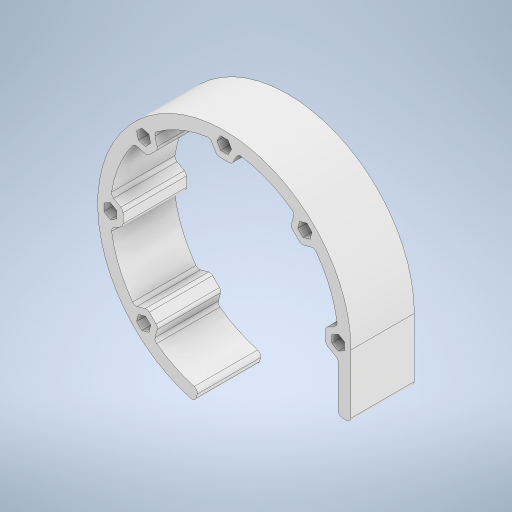
# Autodesk Inventor part: RP_Thigh-cover-connect-1
Saved by Autodesk Inventor 2024.3 (Build 283343000, 343)
## iProperties
Created: 2024-10-20
Part Number: RP_Thigh-cover-connect-1
Material: ABS プラスチック
Document SubType Name: Modeling
Designer: 佐藤智貴
Density: 1.06 g/cm^3
Appearance: 滑らか - 白
Mass: 111.246 g
Surface Area: 471.302 cm^2
Volume: 104.949 cm^3
Author: 佐藤智貴
Autodesk Inventor part; units mm, degrees
ref_plane "YZ Plane" through (0, 0, 0) normal (1, 0, 0) x (0, 1, 0)
ref_plane "XZ Plane" through (0, 0, 0) normal (0, 1, 0) x (-1, 0, 0)
ref_plane "XY Plane" through (0, 0, 0) normal (0, 0, 1) x (1, 0, 0)
sketch "スケッチ1" plane through (0, 0, 0) normal (0, 0, 1) x (1, 0, 0)
  circle A0 centre (0, 0) radius 60
  dimension "d0" = 120
  constraints: 1 centre point, 1 coincident
  measures "d0" diameter of A0
extrude "押し出し1" add sketch "スケッチ1" along normal blind 3
sketch "スケッチ2" plane through (0, 0, 3) normal (0, 0, 1) x (1, 0, 0)
  circle A0 centre (0, 0) radius 46
  line L0 (0, 0) -> (0, 59.211)
  line L1 (0, 0) -> (-21.8609, 52.777)
  line L2 (0, 0) -> (27.8226, 47.8581)
  point P0 (-17.6034, 42.4985)
  point P1 (-42.4985, 17.6034)
  point P2 (-42.4985, -17.6034)
  point P3 (-17.6034, -42.4985)
  point P4 (17.6034, -42.4985)
  point P5 (42.4985, -17.6034)
  point P6 (42.4985, 17.6034)
  point P7 (17.6034, 42.4985)
  dimension "d4" = 92
  dimension "d5" = 22.5
  dimension "d8" = 360
  constraints: 6 end point, 1 coincident, 1 point on line, 1 vertical, 12 other
  measures "d5" angle of L1 L0
hole "穴1" at (-17.6034, 42.4985, 3) at (-42.4985, 17.6034, 3) at (-42.4985, -17.6034, 3) at (-17.6034, -42.4985, 3) at (17.6034, -42.4985, 3) at (42.4985, -17.6034, 3) at (42.4985, 17.6034, 3) at (17.6034, 42.4985, 3) direction (0, 0, -1) diameter 3 end through all
sketch "スケッチ4" plane through (0, 0, 0) normal (0, 0, -1) x (-1, 0, 0)
  line L0 (0, 0) -> (0, -80.557)
  circle A0 centre (0, 0) radius 60 projected
  line L1 (-60, 0) -> (-60, -210)
  line L2 (60, 0) -> (60, -210)
  line L3 (-60, -210) -> (60, -210)
  line L4 (-60, 0) -> (-41.6274, -210)
  line L5 (60, 0) -> (41.6274, -210)
  line L6 (12.7278, -162.7278) -> (60, -210)
  line L7 (19.706, -169.706) -> (-7.6224, -142.3776)
  line L8 (10, -105.557) -> (10, -25)
  circle A1 centre (0, 0) radius 7 projected
  line L9 (10, -177.6776) -> (0, -177.6776)
  line L10 (0, -177.6776) -> (0, -57.7253)
  line L11 (0, -57.7253) -> (10, -57.7253)
  line L12 (10, -57.7253) -> (10, -177.6776)
  point P0 (60, 0)
  point P1 (60, 0)
  point P2 (-59.0885, -10.4189)
  point P3 (-60, -25)
  point P4 (60, -25)
  point P5 (59.0885, -10.4189)
  point P6 (10, -59.1608)
  point P7 (43.1055, -193.1055)
  point P8 (10, -160)
  point P9 (0, -150)
  point P10 (0, -60)
  point P11 (0, -60)
  dimension "d21" = 60
  dimension "d23" = 120
  dimension "d24" = 210
  dimension "d25" = 210
  dimension "d56" = 0
  dimension "d89" = 85
  dimension "d90" = 85
  dimension "d207" = 45
  dimension "d307" = 10
  constraints: 26 end point, 5 point on line, 2 parallel, 2 perpendicular, 1 horizontal, 1 vertical, 3 other
  measures "d21" distance from line of L1 L0.start
  measures "d23" distance between parallel lines of L2 L1
  measures "d24" distance of L2.start L2.end
  measures "d25" distance of L1.start L1.end
  measures "d56" angle of L2 L0
  measures "d89" angle of L3 L5
  measures "d90" angle of L3 L4
  measures "d207" angle of L3 L6
  measures "d307" distance between parallel lines of L8 L0
extrude "押し出し3" add sketch "スケッチ4" against normal blind 3 contours L11 L8 A0 L0 | A0 L8 L12 L7 L10 L0 | L0 L10 L9 L12 L7 L6 L5 L3 L4 A0 | L4 L3 L1 A0 | L7 L12 L9 L10 | L5 L6 L3
sketch "スケッチ17" plane through (0, 0, 3) normal (0, 0, 1) x (1, 0, 0)
  circle A0 centre (0, 0) radius 30
  dimension "d159" = 60
  constraints: 1 centre point, 1 coincident
  measures "d159" diameter of A0
extrude "押し出し10" cut sketch "スケッチ17" against normal blind 10
sketch "スケッチ20" plane through (0, 0, 3) normal (0, 0, 1) x (1, 0, 0)
  line L0 (-60, -210) -> (60, -210) projected
  circle A0 centre (0, 0) radius 30 projected
  line L1 (60, -210) -> (60, 0) projected
  point P0 (1.5, -179.9937)
  point P1 (0, -210)
  point P2 (58.5, -136.6677)
  point P3 (51.5, -210)
  point P4 (48.5, -124.0626)
  point P5 (60, -150)
  dimension "d205" = 180
  dimension "d223" = 58.5
  dimension "d246" = 60
  constraints: 1 midpoint, 1 other
  measures "d205" distance of point (1.5, -179.994) A0.centre
hole "穴8" at (1.5, -179.9937, 3) direction (0, 0, -1) diameter 10 end through all
fillet "フィレット4" radius 10 2 edges at (-60, -210, 1.5) (60, -210, 1.5)
sketch "スケッチ28" plane through (0, 0, 3) normal (0, 0, 1) x (1, 0, 0)
  circle A0 centre (0, 0) radius 60
  circle A1 centre (0, 0) radius 54
  point P0 (0, 54)
  point P1 (-38.1838, 38.1838)
  point P2 (-54, 0)
  point P3 (-38.1838, -38.1838)
  point P4 (0, -54)
  point P5 (38.1838, -38.1838)
  point P6 (54, 0)
  point P7 (38.1838, 38.1838)
  dimension "d309" = 108
  dimension "d308" = 120
  dimension "d312" = 360
  constraints: 1 centre point, 1 coincident, 1 vertical alignment, 11 other
  measures "d308" diameter of A0
hole "穴13" at (-38.1838, 38.1838, 3) at (0, 54, 3) at (38.1838, 38.1838, 3) at (54, 0, 3) at (-38.1838, -38.1838, 3) at (-54, 0, 3) direction (0, 0, -1) diameter 5 end through all
fillet "フィレット11" radius 2.5 1 edges at (-10, -160, 1.5)
sketch "スケッチ32" plane through (0, 0, 3) normal (0, 0, 1) x (1, 0, 0)
  circle A0 centre (-54, 0) radius 2.5 projected
  circle A1 centre (-54, 0) radius 2.5737
  line L0 (-54, 2.5737) -> (-54, 0)
  circle A2 centre (0, 0) radius 60
  circle A3 centre (0, 0) radius 30 projected
  circle A4 centre (0, 0) radius 54
  line L1 (-54, 2.5737) -> (-56.2289, 1.2869)
  line L2 (-56.2289, 1.2869) -> (-56.2289, -1.2869)
  line L3 (-56.2289, -1.2869) -> (-54, -2.5737)
  line L4 (-54, -2.5737) -> (-51.7711, -1.2869)
  line L5 (-51.7711, -1.2869) -> (-51.7711, 1.2869)
  line L6 (-51.7711, 1.2869) -> (-54, 2.5737)
  line L7 (-56.7, 1.5588) -> (-54, 3.1177)
  line L8 (-54, 3.1177) -> (-51.3, 1.5588)
  line L9 (-51.3, 1.5588) -> (-51.3, -1.5588)
  line L10 (-51.3, -1.5588) -> (-54, -3.1177)
  line L11 (-54, -3.1177) -> (-56.7, -1.5588)
  line L12 (-56.7, -1.5588) -> (-56.7, 1.5588)
  line L13 (-48, 3.4641) -> (-54, 6.9282)
  line L14 (-54, 6.9282) -> (-60, 3.4641)
  line L15 (-60, 3.4641) -> (-60, -3.4641)
  line L16 (-60, -3.4641) -> (-54, -6.9282)
  line L17 (-54, -6.9282) -> (-48, -3.4641)
  line L18 (-48, -3.4641) -> (-48, 3.4641)
  line L19 (-43.0827, -33.2848) -> (-44.8759, -39.9769)
  line L20 (-44.8759, -39.9769) -> (-39.9769, -44.8759)
  line L21 (-36.3906, -31.4916) -> (-43.0827, -33.2848)
  line L22 (-31.4916, -36.3906) -> (-36.3906, -31.4916)
  line L23 (-33.2848, -43.0827) -> (-31.4916, -36.3906)
  line L24 (-39.9769, -44.8759) -> (-33.2848, -43.0827)
  line L25 (-35.9792, -40.3883) -> (-38.9907, -41.1952)
  line L26 (-38.9907, -41.1952) -> (-41.1952, -38.9907)
  line L27 (-41.1952, -38.9907) -> (-40.3883, -35.9792)
  line L28 (-40.3883, -35.9792) -> (-37.3768, -35.1723)
  line L29 (-37.3768, -35.1723) -> (-35.1723, -37.3768)
  line L30 (-35.1723, -37.3768) -> (-35.9792, -40.3883)
  line L31 (-6.9282, -54) -> (-3.4641, -60)
  line L32 (-3.4641, -60) -> (3.4641, -60)
  line L33 (-3.4641, -48) -> (-6.9282, -54)
  line L34 (3.4641, -48) -> (-3.4641, -48)
  line L35 (6.9282, -54) -> (3.4641, -48)
  line L36 (3.4641, -60) -> (6.9282, -54)
  line L37 (3.1177, -54) -> (1.5588, -56.7)
  line L38 (1.5588, -56.7) -> (-1.5588, -56.7)
  line L39 (-1.5588, -56.7) -> (-3.1177, -54)
  line L40 (-3.1177, -54) -> (-1.5588, -51.3)
  line L41 (-1.5588, -51.3) -> (1.5588, -51.3)
  line L42 (1.5588, -51.3) -> (3.1177, -54)
  line L43 (33.2848, -43.0827) -> (39.9769, -44.8759)
  line L44 (39.9769, -44.8759) -> (44.8759, -39.9769)
  line L45 (31.4916, -36.3906) -> (33.2848, -43.0827)
  line L46 (36.3906, -31.4916) -> (31.4916, -36.3906)
  line L47 (43.0827, -33.2848) -> (36.3906, -31.4916)
  line L48 (44.8759, -39.9769) -> (43.0827, -33.2848)
  line L49 (40.3883, -35.9792) -> (41.1952, -38.9907)
  line L50 (41.1952, -38.9907) -> (38.9907, -41.1952)
  line L51 (38.9907, -41.1952) -> (35.9792, -40.3883)
  line L52 (35.9792, -40.3883) -> (35.1723, -37.3768)
  line L53 (35.1723, -37.3768) -> (37.3768, -35.1723)
  line L54 (37.3768, -35.1723) -> (40.3883, -35.9792)
  line L55 (54, -6.9282) -> (60, -3.4641)
  line L56 (60, -3.4641) -> (60, 3.4641)
  line L57 (48, -3.4641) -> (54, -6.9282)
  line L58 (48, 3.4641) -> (48, -3.4641)
  line L59 (54, 6.9282) -> (48, 3.4641)
  line L60 (60, 3.4641) -> (54, 6.9282)
  line L61 (54, 3.1177) -> (56.7, 1.5588)
  line L62 (56.7, 1.5588) -> (56.7, -1.5588)
  line L63 (56.7, -1.5588) -> (54, -3.1177)
  line L64 (54, -3.1177) -> (51.3, -1.5588)
  line L65 (51.3, -1.5588) -> (51.3, 1.5588)
  line L66 (51.3, 1.5588) -> (54, 3.1177)
  line L67 (43.0827, 33.2848) -> (44.8759, 39.9769)
  line L68 (44.8759, 39.9769) -> (39.9769, 44.8759)
  line L69 (36.3906, 31.4916) -> (43.0827, 33.2848)
  line L70 (31.4916, 36.3906) -> (36.3906, 31.4916)
  line L71 (33.2848, 43.0827) -> (31.4916, 36.3906)
  line L72 (39.9769, 44.8759) -> (33.2848, 43.0827)
  line L73 (35.9792, 40.3883) -> (38.9907, 41.1952)
  line L74 (38.9907, 41.1952) -> (41.1952, 38.9907)
  line L75 (41.1952, 38.9907) -> (40.3883, 35.9792)
  line L76 (40.3883, 35.9792) -> (37.3768, 35.1723)
  line L77 (37.3768, 35.1723) -> (35.1723, 37.3768)
  line L78 (35.1723, 37.3768) -> (35.9792, 40.3883)
  line L79 (6.9282, 54) -> (3.4641, 60)
  line L80 (3.4641, 60) -> (-3.4641, 60)
  line L81 (3.4641, 48) -> (6.9282, 54)
  line L82 (-3.4641, 48) -> (3.4641, 48)
  line L83 (-6.9282, 54) -> (-3.4641, 48)
  line L84 (-3.4641, 60) -> (-6.9282, 54)
  line L85 (-3.1177, 54) -> (-1.5588, 56.7)
  line L86 (-1.5588, 56.7) -> (1.5588, 56.7)
  line L87 (1.5588, 56.7) -> (3.1177, 54)
  line L88 (3.1177, 54) -> (1.5588, 51.3)
  line L89 (1.5588, 51.3) -> (-1.5588, 51.3)
  line L90 (-1.5588, 51.3) -> (-3.1177, 54)
  line L91 (-33.2848, 43.0827) -> (-39.9769, 44.8759)
  line L92 (-39.9769, 44.8759) -> (-44.8759, 39.9769)
  line L93 (-31.4916, 36.3906) -> (-33.2848, 43.0827)
  line L94 (-36.3906, 31.4916) -> (-31.4916, 36.3906)
  line L95 (-43.0827, 33.2848) -> (-36.3906, 31.4916)
  line L96 (-44.8759, 39.9769) -> (-43.0827, 33.2848)
  line L97 (-40.3883, 35.9792) -> (-41.1952, 38.9907)
  line L98 (-41.1952, 38.9907) -> (-38.9907, 41.1952)
  line L99 (-38.9907, 41.1952) -> (-35.9792, 40.3883)
  line L100 (-35.9792, 40.3883) -> (-35.1723, 37.3768)
  line L101 (-35.1723, 37.3768) -> (-37.3768, 35.1723)
  line L102 (-37.3768, 35.1723) -> (-40.3883, 35.9792)
  line L103 (-10, -59.1608) -> (-10, -158.9645) projected
  line L104 (-10, -59.1608) -> (-4, -59.1608)
  line L105 (-4, -59.1608) -> (-4, -158.9645)
  line L106 (-4, -158.9645) -> (-10, -158.9645)
  line L107 (-10, -158.9645) -> (-10, -59.1608)
  line L108 (60, 0) -> (54, 0)
  line L109 (54, 0) -> (54, -158.9645)
  line L110 (60, -158.9645) -> (60, 0)
  line L111 (-10, -59.1608) -> (-4, -59.1608)
  line L112 (-4, -59.1608) -> (-4, -48.9282)
  line L113 (-4, -48.9282) -> (-10, -48.9282)
  line L114 (-10, -48.9282) -> (-10, -59.1608)
  circle A5 centre (-4, -69.1608) radius 2.5
  circle A6 centre (-4, -69.1608) radius 3.2562
  line L115 (-4, -65.9046) -> (-4, -69.1608)
  line L116 (-4, -65.9046) -> (-6.82, -67.5327)
  line L117 (-6.82, -67.5327) -> (-6.82, -70.7889)
  line L118 (-6.82, -70.7889) -> (-4, -72.417)
  line L119 (-4, -72.417) -> (-1.18, -70.7889)
  line L120 (-1.18, -70.7889) -> (-1.18, -67.5327)
  line L121 (-1.18, -67.5327) -> (-4, -65.9046)
  line L122 (-6.7, -67.602) -> (-4, -66.0431)
  line L123 (-4, -66.0431) -> (-1.3, -67.602)
  line L124 (-1.3, -67.602) -> (-1.3, -70.7196)
  line L125 (-1.3, -70.7196) -> (-4, -72.2785)
  line L126 (-4, -72.2785) -> (-6.7, -70.7196)
  line L127 (-6.7, -70.7196) -> (-6.7, -67.602)
  line L128 (2, -65.6967) -> (-4, -62.2326)
  line L129 (-4, -62.2326) -> (-10, -65.6967)
  line L130 (-10, -65.6967) -> (-10, -72.6249)
  line L131 (-10, -72.6249) -> (-4, -76.089)
  line L132 (-4, -76.089) -> (2, -72.6249)
  line L133 (2, -72.6249) -> (2, -65.6967)
  line L134 (-4, -102.2326) -> (-10, -105.6967)
  line L135 (2, -105.6967) -> (-4, -102.2326)
  line L136 (2, -112.6249) -> (2, -105.6967)
  line L137 (-4, -116.089) -> (2, -112.6249)
  line L138 (-10, -112.6249) -> (-4, -116.089)
  line L139 (-4, -112.2785) -> (-6.7, -110.7196)
  line L140 (-1.3, -110.7196) -> (-4, -112.2785)
  line L141 (-1.3, -107.602) -> (-1.3, -110.7196)
  line L142 (-4, -106.0431) -> (-1.3, -107.602)
  line L143 (-6.7, -107.602) -> (-4, -106.0431)
  line L144 (-6.7, -110.7196) -> (-6.7, -107.602)
  line L145 (60, -36.5359) -> (54, -33.0718)
  line L146 (60, -43.4641) -> (60, -36.5359)
  line L147 (54, -46.9282) -> (60, -43.4641)
  line L148 (48, -43.4641) -> (54, -46.9282)
  line L149 (48, -36.5359) -> (48, -43.4641)
  line L150 (54, -33.0718) -> (48, -36.5359)
  line L151 (51.3, -38.4412) -> (54, -36.8823)
  line L152 (51.3, -41.5588) -> (51.3, -38.4412)
  line L153 (54, -43.1177) -> (51.3, -41.5588)
  line L154 (56.7, -41.5588) -> (54, -43.1177)
  line L155 (56.7, -38.4412) -> (56.7, -41.5588)
  line L156 (54, -36.8823) -> (56.7, -38.4412)
  line L157 (-4, -142.2326) -> (-10, -145.6967)
  line L158 (2, -145.6967) -> (-4, -142.2326)
  line L159 (2, -152.6249) -> (2, -145.6967)
  line L160 (-4, -156.089) -> (2, -152.6249)
  line L161 (-10, -152.6249) -> (-4, -156.089)
  line L162 (-4, -152.2785) -> (-6.7, -150.7196)
  line L163 (-1.3, -150.7196) -> (-4, -152.2785)
  line L164 (-1.3, -147.602) -> (-1.3, -150.7196)
  line L165 (-4, -146.0431) -> (-1.3, -147.602)
  line L166 (-6.7, -147.602) -> (-4, -146.0431)
  line L167 (-6.7, -150.7196) -> (-6.7, -147.602)
  line L168 (60, -76.5359) -> (54, -73.0718)
  line L169 (60, -83.4641) -> (60, -76.5359)
  line L170 (54, -86.9282) -> (60, -83.4641)
  line L171 (48, -83.4641) -> (54, -86.9282)
  line L172 (48, -76.5359) -> (48, -83.4641)
  line L173 (54, -73.0718) -> (48, -76.5359)
  line L174 (51.3, -78.4412) -> (54, -76.8823)
  line L175 (51.3, -81.5588) -> (51.3, -78.4412)
  line L176 (54, -83.1177) -> (51.3, -81.5588)
  line L177 (56.7, -81.5588) -> (54, -83.1177)
  line L178 (56.7, -78.4412) -> (56.7, -81.5588)
  line L179 (54, -76.8823) -> (56.7, -78.4412)
  line L180 (54, -113.0718) -> (48, -116.5359)
  line L181 (60, -116.5359) -> (54, -113.0718)
  line L182 (48, -116.5359) -> (48, -123.4641)
  line L183 (48, -123.4641) -> (54, -126.9282)
  line L184 (54, -126.9282) -> (60, -123.4641)
  line L185 (54, -116.8823) -> (56.7, -118.4412)
  line L186 (51.3, -118.4412) -> (54, -116.8823)
  line L187 (56.7, -118.4412) -> (56.7, -121.5588)
  line L188 (56.7, -121.5588) -> (54, -123.1177)
  line L189 (54, -123.1177) -> (51.3, -121.5588)
  line L190 (51.3, -121.5588) -> (51.3, -118.4412)
  line L191 (54, -153.0718) -> (48, -156.5359)
  line L192 (60, -156.5359) -> (54, -153.0718)
  line L193 (48, -156.5359) -> (48, -163.4641)
  line L194 (48, -163.4641) -> (54, -166.9282)
  line L195 (54, -166.9282) -> (60, -163.4641)
  line L196 (54, -156.8823) -> (56.7, -158.4412)
  line L197 (51.3, -158.4412) -> (54, -156.8823)
  line L198 (56.7, -158.4412) -> (56.7, -161.5588)
  line L199 (56.7, -161.5588) -> (54, -163.1177)
  line L200 (54, -163.1177) -> (51.3, -161.5588)
  line L201 (51.3, -161.5588) -> (51.3, -158.4412)
  line L202 (54, -158.9645) -> (54, -174.0118)
  line L203 (54, -174.0118) -> (60, -174.0118)
  line L204 (60, -174.0118) -> (60, -158.9645)
  line L205 (54, -66.9282) -> (60, -63.4641)
  line L206 (48, -63.4641) -> (54, -66.9282)
  line L207 (48, -56.5359) -> (48, -63.4641)
  line L208 (54, -53.0718) -> (48, -56.5359)
  line L209 (60, -56.5359) -> (54, -53.0718)
  line L210 (56.7, -58.4412) -> (56.7, -61.5588)
  line L211 (54, -56.8823) -> (56.7, -58.4412)
  line L212 (51.3, -58.4412) -> (54, -56.8823)
  line L213 (51.3, -61.5588) -> (51.3, -58.4412)
  line L214 (54, -63.1177) -> (51.3, -61.5588)
  line L215 (56.7, -61.5588) -> (54, -63.1177)
  line L216 (54, -86.9282) -> (60, -83.4641)
  line L217 (48, -83.4641) -> (54, -86.9282)
  line L218 (48, -76.5359) -> (48, -83.4641)
  line L219 (54, -73.0718) -> (48, -76.5359)
  line L220 (60, -76.5359) -> (54, -73.0718)
  line L221 (56.7, -78.4412) -> (56.7, -81.5588)
  line L222 (54, -76.8823) -> (56.7, -78.4412)
  line L223 (51.3, -78.4412) -> (54, -76.8823)
  line L224 (51.3, -81.5588) -> (51.3, -78.4412)
  line L225 (54, -83.1177) -> (51.3, -81.5588)
  line L226 (56.7, -81.5588) -> (54, -83.1177)
  line L227 (54, -106.9282) -> (60, -103.4641)
  line L228 (48, -103.4641) -> (54, -106.9282)
  line L229 (48, -96.5359) -> (48, -103.4641)
  line L230 (54, -93.0718) -> (48, -96.5359)
  line L231 (60, -96.5359) -> (54, -93.0718)
  line L232 (56.7, -98.4412) -> (56.7, -101.5588)
  line L233 (54, -96.8823) -> (56.7, -98.4412)
  line L234 (51.3, -98.4412) -> (54, -96.8823)
  line L235 (51.3, -101.5588) -> (51.3, -98.4412)
  line L236 (54, -103.1177) -> (51.3, -101.5588)
  line L237 (56.7, -101.5588) -> (54, -103.1177)
  line L238 (54, -126.9282) -> (60, -123.4641)
  line L239 (48, -123.4641) -> (54, -126.9282)
  line L240 (48, -116.5359) -> (48, -123.4641)
  line L241 (54, -113.0718) -> (48, -116.5359)
  line L242 (60, -116.5359) -> (54, -113.0718)
  line L243 (56.7, -118.4412) -> (56.7, -121.5588)
  line L244 (54, -116.8823) -> (56.7, -118.4412)
  line L245 (51.3, -118.4412) -> (54, -116.8823)
  line L246 (51.3, -121.5588) -> (51.3, -118.4412)
  line L247 (54, -123.1177) -> (51.3, -121.5588)
  line L248 (56.7, -121.5588) -> (54, -123.1177)
  line L249 (54, -146.9282) -> (60, -143.4641)
  line L250 (48, -143.4641) -> (54, -146.9282)
  line L251 (48, -136.5359) -> (48, -143.4641)
  line L252 (54, -133.0718) -> (48, -136.5359)
  line L253 (60, -136.5359) -> (54, -133.0718)
  line L254 (56.7, -138.4412) -> (56.7, -141.5588)
  line L255 (54, -136.8823) -> (56.7, -138.4412)
  line L256 (51.3, -138.4412) -> (54, -136.8823)
  line L257 (51.3, -141.5588) -> (51.3, -138.4412)
  line L258 (54, -143.1177) -> (51.3, -141.5588)
  line L259 (56.7, -141.5588) -> (54, -143.1177)
  line L260 (54, -166.9282) -> (60, -163.4641)
  line L261 (48, -163.4641) -> (54, -166.9282)
  line L262 (48, -156.5359) -> (48, -163.4641)
  line L263 (54, -153.0718) -> (48, -156.5359)
  line L264 (60, -156.5359) -> (54, -153.0718)
  line L265 (56.7, -158.4412) -> (56.7, -161.5588)
  line L266 (54, -156.8823) -> (56.7, -158.4412)
  line L267 (51.3, -158.4412) -> (54, -156.8823)
  line L268 (51.3, -161.5588) -> (51.3, -158.4412)
  line L269 (54, -163.1177) -> (51.3, -161.5588)
  line L270 (56.7, -161.5588) -> (54, -163.1177)
  line L271 (54, -186.9282) -> (60, -183.4641)
  line L272 (48, -183.4641) -> (54, -186.9282)
  line L273 (48, -176.5359) -> (48, -183.4641)
  line L274 (54, -173.0718) -> (48, -176.5359)
  line L275 (60, -176.5359) -> (54, -173.0718)
  line L276 (56.7, -178.4412) -> (56.7, -181.5588)
  line L277 (54, -176.8823) -> (56.7, -178.4412)
  line L278 (51.3, -178.4412) -> (54, -176.8823)
  line L279 (51.3, -181.5588) -> (51.3, -178.4412)
  line L280 (54, -183.1177) -> (51.3, -181.5588)
  line L281 (56.7, -181.5588) -> (54, -183.1177)
  line L282 (2, -95.6967) -> (-4, -92.2326)
  line L283 (-4, -92.2326) -> (-10, -95.6967)
  line L284 (-10, -102.6249) -> (-4, -106.089)
  line L285 (-4, -106.089) -> (2, -102.6249)
  line L286 (2, -102.6249) -> (2, -95.6967)
  line L287 (-1.3, -97.602) -> (-1.3, -100.7196)
  line L288 (-4, -96.0431) -> (-1.3, -97.602)
  line L289 (-6.7, -97.602) -> (-4, -96.0431)
  line L290 (-6.7, -100.7196) -> (-6.7, -97.602)
  line L291 (-4, -102.2785) -> (-6.7, -100.7196)
  line L292 (-1.3, -100.7196) -> (-4, -102.2785)
  line L293 (2, -125.6967) -> (-4, -122.2326)
  line L294 (-4, -122.2326) -> (-10, -125.6967)
  line L295 (-10, -132.6249) -> (-4, -136.089)
  line L296 (-4, -136.089) -> (2, -132.6249)
  line L297 (2, -132.6249) -> (2, -125.6967)
  line L298 (-1.3, -127.602) -> (-1.3, -130.7196)
  line L299 (-4, -126.0431) -> (-1.3, -127.602)
  line L300 (-6.7, -127.602) -> (-4, -126.0431)
  line L301 (-6.7, -130.7196) -> (-6.7, -127.602)
  line L302 (-4, -132.2785) -> (-6.7, -130.7196)
  line L303 (-1.3, -130.7196) -> (-4, -132.2785)
  line L304 (-51, 1.7321) -> (-54, 3.4641)
  line L305 (-54, 3.4641) -> (-57, 1.7321)
  line L306 (-57, 1.7321) -> (-57, -1.7321)
  line L307 (-57, -1.7321) -> (-54, -3.4641)
  line L308 (-54, -3.4641) -> (-51, -1.7321)
  line L309 (-51, -1.7321) -> (-51, 1.7321)
  point P0 (-42.619, -33.1605)
  point P1 (-53.5842, -6.6882)
  point P2 (-53.5842, 6.6882)
  point P3 (-42.619, 33.1605)
  point P4 (-33.1605, 42.619)
  point P5 (-6.6882, 53.5842)
  point P6 (6.6882, 53.5842)
  point P7 (33.1605, 42.619)
  point P8 (42.619, 33.1605)
  point P9 (53.5842, 6.6882)
  point P10 (60, 0)
  point P11 (-4, -59.8665)
  point P12 (-3.5239, -59.8964)
  point P13 (-6.6882, -53.5842)
  point P14 (-33.1605, -42.619)
  point P15 (-44.8449, 39.8614)
  point P16 (-59.8964, 3.5239)
  point P17 (60, -40)
  point P18 (60, -80)
  point P19 (54, -156.8823)
  point P20 (59.8964, 3.5239)
  point P21 (-4, -76.089)
  point P22 (-4, -53.8516)
  point P23 (-39.8614, -44.8449)
  point P24 (54, -163.1177)
  point P25 (54, -156.8823)
  point P26 (54, -163.1177)
  point P27 (39.8614, 44.8449)
  point P28 (56.7, 0)
  point P29 (56.7, -160)
  point P30 (57, 0)
  point P31 (56.7, -40)
  point P32 (56.7, -80)
  point P33 (-10, -53.066)
  point P34 (53.5842, -6.6882)
  point P35 (53.9128, -3.0674)
  point P36 (54, -3.1177)
  point P37 (54, -3.1177)
  dimension "d410" = 6
  dimension "d413" = 360
  dimension "d415" = 5.4
  dimension "d417" = 12
  dimension "d420" = 360
  dimension "d422" = 6
  dimension "d423" = 6
  dimension "d430" = 360
  dimension "d431" = 5.4
  dimension "d432" = 12
  dimension "d433" = 0
  dimension "d434" = 10
  dimension "d437" = 40
  dimension "d444" = 40
  dimension "d451" = 20
  dimension "d457" = 160
  dimension "d458" = 40
  dimension "d459" = 40
  dimension "d465" = 30
  dimension "d470" = 6
  constraints: 618 end point, 27 parallel, 8 vertical, 6 midpoint, 4 coincident, 3 horizontal, 3 perpendicular, 2 point on line, 2 vertical alignment, 1 centre point, 590 other
  measures "d415" distance between parallel lines of L9 L12
  measures "d417" distance between parallel lines of L15 L18
  measures "d422" distance of L103.start L104.end
  measures "d423" distance between parallel lines of L110 L109
  measures "d431" distance between parallel lines of L124 L127
  measures "d432" distance between parallel lines of L130 L133
  measures "d433" distance from line of L105 point (-4, -69.161)
  measures "d434" distance from line of L104 point (-4, -69.161)
  measures "d437" distance of L129.start L134.start
  measures "d444" distance of L168.end L180.start
  measures "d451" distance of L147.start L205.start
  measures "d457" distance of point (56.7, 0) point (56.7, -160)
  measures "d458" vertical distance of point (57, 0) point (56.7, -40)
  measures "d459" distance of point (56.7, -80) point (56.7, -40)
  measures "d465" distance of L128.start L282.start
  measures "d470" distance from line of L309 L305.end
extrude "押し出し17" add sketch "スケッチ32" along normal blind 32 contours L8 L7 L12 L11 L10 A4 L308 L307 L306 L305 L304 | A4 L304 L309 L308 L10 L9 L8 | L304 L305 L306 L307 L308 A4 L17 L16 A2 L14 L13 | A4 L13 L18 L17 L308 L309 L304 | L13 L14 A2 L96 L95 A4 | A4 L21 L19 A2 L16 L17 | L95 L96 A2 L91 L93 A4 L100 L99 L98 L97 L102 | A4 L102 L101 L100 L93 L94 L95 | L21 L22 L23 A4 L30 L29 L28 | A4 L28 L27 L26 L25 L30 L23 L24 A2 L19 L21 | L93 L91 A2 L84 L83 A4 | A4 L114 A2 L24 L23 | L83 L84 A2 L79 L81 A4 L88 L87 L86 L85 L90 | A4 L90 L89 L88 L81 L82 L83 | A4 L33 L31 L112 L104 L114 | A4 L112 L31 L33 | L104 L105 A2 | A2 L105 L129 L103 | L129 L105 A6 L131 L103 | L81 L79 A2 L72 L71 A4 | L128 L133 L132 L105 A6 | L131 L105 L283 L103 | L71 L72 A2 L67 L69 A4 L76 L75 L74 L73 L78 | A4 L78 L77 L76 L69 L70 L71 | L121 L120 L119 L105 L125 L124 L123 | L116 A6 | L105 L122 L127 L126 L118 L117 L116 | A6 L121 | L283 L105 L289 L290 L291 L134 L284 L103 | A6 L120 | L117 A6 | L284 L134 L103 | L282 L286 L285 L135 L292 L287 L288 L105 | L119 A6 | A6 L118 | A2 L60 L59 A4 L69 L67 | L134 L284 L143 L144 L139 L105 L138 L103 | L134 L291 L105 L143 L284 | A2 L108 L62 L61 L66 A4 L59 L60 | L138 L105 L294 L103 | L284 L105 L139 L144 L143 | L143 L105 L284 | A4 L66 L65 L64 L57 L58 L59 | L56 L55 A2 | A2 L55 L109 L63 L62 L108 | L294 L105 L300 L301 L302 L295 L103 | L292 L135 L285 L142 L105 | L142 L285 L105 | L55 L110 L145 L109 A2 | A2 L109 L55 | L293 L297 L296 L105 L303 L298 L299 | L57 A4 L64 L109 | L110 L147 L109 L154 L155 L156 L145 | L109 L151 L152 L153 L148 L149 L150 | L110 L209 L109 L147 | L110 L205 L109 L215 L210 L211 L209 | L110 L168 L109 L205 | L110 L170 L109 L177 L178 L179 L168 | L211 L210 L215 L109 | L110 L231 L109 L170 | L109 L174 L175 L176 L171 L172 L173 | L110 L227 L109 L237 L232 L233 L231 | L110 L181 L109 L227 | L110 L184 L109 L188 L187 L185 L181 | L233 L232 L237 L109 | L110 L253 L109 L184 | L109 L186 L190 L189 L183 L182 L180 | L110 L249 L109 L259 L254 L255 L253 | L110 L192 L109 L249 | L110 L204 L195 L202 L199 L198 L196 L109 L192 | L255 L254 L259 L109 | L109 L197 L201 L200 L202 L194 L193 L191
sketch "スケッチ33" plane through (0, 0, 0) normal (0, 0, -1) x (-1, 0, 0)
  line L0 (-123.2071, 75.0132) -> (142.9686, 75.0132)
  line L1 (142.9686, 75.0132) -> (142.9686, -231.089)
  line L2 (142.9686, -231.089) -> (-123.2071, -231.089)
  line L3 (-123.2071, -231.089) -> (-123.2071, 75.0132)
  point P0 (0, 0)
  constraints: 8 end point, 2 parallel, 1 horizontal, 1 perpendicular
extrude "押し出し18" cut sketch "スケッチ33" against normal blind 5
fillet "フィレット15" radius 5 2 edges at (-4, -53.8516, 20) (-10, -59.1608, 20)
fillet "フィレット16" radius 2 22 edges at (-4, -76.089, 20) (2, -72.6249, 20) (2, -65.6967, 20) (-4, -62.2326, 20) (48, -163.4641, 20) (48, -156.5359, 20) (54, -153.0718, 20) (54, -166.9282, 20) (60, -163.4641, 20) (54, -126.9282, 20) (48, -123.4641, 20) (48, -116.5359, 20) (54, -113.0718, 20) (2, -102.6249, 20) (-4, -106.089, 20) (2, -95.6967, 20) (-4, -92.2326, 20) (-10, -132.6249, 20) (-4, -136.089, 20) (2, -132.6249, 20) (-4, -122.2326, 20) (2, -125.6967, 20)
fillet "フィレット17" radius 2 32 edges at (48, -76.5359, 20) (48, -83.4641, 20) (54, -86.9282, 20) (54, -73.0718, 20) (54, -46.9282, 20) (48, -43.4641, 20) (48, -36.5359, 20) (54, -6.9282, 20) (48, -3.4641, 20) (48, 3.4641, 20) (53.5842, 6.6882, 20) (42.619, 33.1605, 20) (36.3906, 31.4916, 20) (31.4916, 36.3906, 20) (33.1605, 42.619, 20) (6.6882, 53.5842, 20) (3.4641, 48, 20) (-3.4641, 48, 20) (-6.6882, 53.5842, 20) (-42.619, 33.1605, 20) (-36.3906, 31.4916, 20) (-31.4916, 36.3906, 20) (-48, -3.4641, 20) (-48, 3.4641, 20) (-33.1605, 42.619, 20) (-53.5842, 6.6882, 20) (-42.619, -33.1605, 20) (-36.3906, -31.4916, 20) (-31.4916, -36.3906, 20) (-33.1605, -42.619, 20) (-53.5842, -6.6882, 20) (54, -33.0718, 20)
sketch "スケッチ34" plane through (0, 0, 35) normal (0, 0, 1) x (1, 0, 0)
  line L0 (-54, 3.1177) -> (-51.3, 1.5588) projected
  line L1 (-56.7, 1.5588) -> (-54, 3.1177) projected
  line L2 (-54, 3.1177) -> (-56.7, 1.5588)
  line L3 (-54, -3.1177) -> (-56.7, -1.5588) projected
  line L4 (-56.7, 1.5588) -> (-56.7, -1.5588)
  line L5 (-56.7, -1.5588) -> (-54, -3.1177)
  line L6 (-54, -3.1177) -> (-51.3, -1.5588)
  line L7 (-51.3, 1.5588) -> (-54, 3.1177)
  line L8 (-51.3, 1.5588) -> (-51.3, -1.5588) projected
  line L9 (-51.3, 1.5588) -> (-51.3, -1.5588)
  line L10 (-57, -1.7321) -> (-57, 1.7321)
  line L11 (-57, 1.7321) -> (-54, 3.4641)
  line L12 (-54, 3.4641) -> (-51, 1.7321)
  line L13 (-51, 1.7321) -> (-51, -1.7321)
  line L14 (-51, -1.7321) -> (-54, -3.4641)
  line L15 (-54, -3.4641) -> (-57, -1.7321)
  circle A0 centre (0, 0) radius 54
  line L16 (-34.8377, -37.2872) -> (-35.7343, -40.6333)
  line L17 (-35.7343, -40.6333) -> (-39.0803, -41.5298)
  line L18 (-39.0803, -41.5298) -> (-41.5298, -39.0803)
  line L19 (-41.5298, -39.0803) -> (-40.6333, -35.7343)
  line L20 (-40.6333, -35.7343) -> (-37.2872, -34.8377)
  line L21 (-37.2872, -34.8377) -> (-34.8377, -37.2872)
  line L22 (1.7321, -51) -> (3.4641, -54)
  line L23 (3.4641, -54) -> (1.7321, -57)
  line L24 (1.7321, -57) -> (-1.7321, -57)
  line L25 (-1.7321, -57) -> (-3.4641, -54)
  line L26 (-3.4641, -54) -> (-1.7321, -51)
  line L27 (-1.7321, -51) -> (1.7321, -51)
  line L28 (37.2872, -34.8377) -> (40.6333, -35.7343)
  line L29 (40.6333, -35.7343) -> (41.5298, -39.0803)
  line L30 (41.5298, -39.0803) -> (39.0803, -41.5298)
  line L31 (39.0803, -41.5298) -> (35.7343, -40.6333)
  line L32 (35.7343, -40.6333) -> (34.8377, -37.2872)
  line L33 (34.8377, -37.2872) -> (37.2872, -34.8377)
  line L34 (51, 1.7321) -> (54, 3.4641)
  line L35 (54, 3.4641) -> (57, 1.7321)
  line L36 (57, 1.7321) -> (57, -1.7321)
  line L37 (57, -1.7321) -> (54, -3.4641)
  line L38 (54, -3.4641) -> (51, -1.7321)
  line L39 (51, -1.7321) -> (51, 1.7321)
  line L40 (34.8377, 37.2872) -> (35.7343, 40.6333)
  line L41 (35.7343, 40.6333) -> (39.0803, 41.5298)
  line L42 (39.0803, 41.5298) -> (41.5298, 39.0803)
  line L43 (41.5298, 39.0803) -> (40.6333, 35.7343)
  line L44 (40.6333, 35.7343) -> (37.2872, 34.8377)
  line L45 (37.2872, 34.8377) -> (34.8377, 37.2872)
  line L46 (-1.7321, 51) -> (-3.4641, 54)
  line L47 (-3.4641, 54) -> (-1.7321, 57)
  line L48 (-1.7321, 57) -> (1.7321, 57)
  line L49 (1.7321, 57) -> (3.4641, 54)
  line L50 (3.4641, 54) -> (1.7321, 51)
  line L51 (1.7321, 51) -> (-1.7321, 51)
  line L52 (-37.2872, 34.8377) -> (-40.6333, 35.7343)
  line L53 (-40.6333, 35.7343) -> (-41.5298, 39.0803)
  line L54 (-41.5298, 39.0803) -> (-39.0803, 41.5298)
  line L55 (-39.0803, 41.5298) -> (-35.7343, 40.6333)
  line L56 (-35.7343, 40.6333) -> (-34.8377, 37.2872)
  line L57 (-34.8377, 37.2872) -> (-37.2872, 34.8377)
  line L58 (-40.3883, -35.9792) -> (-41.1952, -38.9907)
  line L59 (-37.3768, -35.1723) -> (-40.3883, -35.9792)
  line L60 (-37.3768, -35.1723) -> (-35.1723, -37.3768)
  line L61 (-35.9792, -40.3883) -> (-35.1723, -37.3768)
  line L62 (-38.9907, -41.1952) -> (-35.9792, -40.3883)
  line L63 (-41.1952, -38.9907) -> (-38.9907, -41.1952)
  line L64 (-3.1177, -54) -> (-1.5588, -56.7)
  line L65 (-1.5588, -51.3) -> (-3.1177, -54)
  line L66 (-1.5588, -51.3) -> (1.5588, -51.3)
  line L67 (3.1177, -54) -> (1.5588, -51.3)
  line L68 (1.5588, -56.7) -> (3.1177, -54)
  line L69 (-1.5588, -56.7) -> (1.5588, -56.7)
  line L70 (35.9792, -40.3883) -> (38.9907, -41.1952)
  line L71 (35.1723, -37.3768) -> (35.9792, -40.3883)
  line L72 (35.1723, -37.3768) -> (37.3768, -35.1723)
  line L73 (40.3883, -35.9792) -> (37.3768, -35.1723)
  line L74 (41.1952, -38.9907) -> (40.3883, -35.9792)
  line L75 (38.9907, -41.1952) -> (41.1952, -38.9907)
  line L76 (54, -3.1177) -> (56.7, -1.5588)
  line L77 (51.3, -1.5588) -> (54, -3.1177)
  line L78 (51.3, -1.5588) -> (51.3, 1.5588)
  line L79 (54, 3.1177) -> (51.3, 1.5588)
  line L80 (56.7, 1.5588) -> (54, 3.1177)
  line L81 (56.7, -1.5588) -> (56.7, 1.5588)
  line L82 (40.3883, 35.9792) -> (41.1952, 38.9907)
  line L83 (37.3768, 35.1723) -> (40.3883, 35.9792)
  line L84 (37.3768, 35.1723) -> (35.1723, 37.3768)
  line L85 (35.9792, 40.3883) -> (35.1723, 37.3768)
  line L86 (38.9907, 41.1952) -> (35.9792, 40.3883)
  line L87 (41.1952, 38.9907) -> (38.9907, 41.1952)
  line L88 (3.1177, 54) -> (1.5588, 56.7)
  line L89 (1.5588, 51.3) -> (3.1177, 54)
  line L90 (1.5588, 51.3) -> (-1.5588, 51.3)
  line L91 (-3.1177, 54) -> (-1.5588, 51.3)
  line L92 (-1.5588, 56.7) -> (-3.1177, 54)
  line L93 (1.5588, 56.7) -> (-1.5588, 56.7)
  line L94 (-35.9792, 40.3883) -> (-38.9907, 41.1952)
  line L95 (-35.1723, 37.3768) -> (-35.9792, 40.3883)
  line L96 (-35.1723, 37.3768) -> (-37.3768, 35.1723)
  line L97 (-40.3883, 35.9792) -> (-37.3768, 35.1723)
  line L98 (-41.1952, 38.9907) -> (-40.3883, 35.9792)
  line L99 (-38.9907, 41.1952) -> (-41.1952, 38.9907)
  line L100 (-4, -66.0431) -> (-1.3, -67.602) projected
  line L101 (-6.7, -67.602) -> (-4, -66.0431) projected
  line L102 (-4, -66.0431) -> (-6.7, -67.602)
  line L103 (-6.7, -70.7196) -> (-6.7, -67.602) projected
  line L104 (-6.7, -67.602) -> (-6.7, -70.7196)
  line L105 (-4, -72.2785) -> (-6.7, -70.7196) projected
  line L106 (-6.7, -70.7196) -> (-4, -72.2785)
  line L107 (-4, -72.2785) -> (-1.3, -70.7196)
  line L108 (-1.3, -67.602) -> (-1.3, -70.7196) projected
  line L109 (-1.3, -70.7196) -> (-1.3, -67.602)
  line L110 (-1.3, -67.602) -> (-4, -66.0431)
  line L111 (-1, -70.8928) -> (-4, -72.6249)
  line L112 (-4, -72.6249) -> (-7, -70.8928)
  line L113 (-7, -70.8928) -> (-7, -67.4287)
  line L114 (-7, -67.4287) -> (-4, -65.6967)
  line L115 (-4, -65.6967) -> (-1, -67.4287)
  line L116 (-1, -67.4287) -> (-1, -70.8928)
  line L117 (-4, -102.2785) -> (-6.7, -100.7196) projected
  line L118 (-4, -72.6249) -> (-4, -102.2785)
  line L119 (-7, -97.4287) -> (-4, -95.6967)
  line L120 (-4, -95.6967) -> (-1, -97.4287)
  line L121 (-1.3, -97.602) -> (-4, -96.0431)
  line L122 (-4, -96.0431) -> (-6.7, -97.602)
  line L123 (-7, -100.8928) -> (-7, -97.4287)
  line L124 (-6.7, -97.602) -> (-6.7, -100.7196)
  line L125 (-1.3, -100.7196) -> (-1.3, -97.602)
  line L126 (-1, -97.4287) -> (-1, -100.8928)
  line L127 (-1, -100.8928) -> (-4, -102.6249)
  line L128 (-4, -102.2785) -> (-1.3, -100.7196)
  line L129 (-6.7, -100.7196) -> (-4, -102.2785)
  line L130 (-4, -102.6249) -> (-7, -100.8928)
  line L131 (-7, -127.4287) -> (-4, -125.6967)
  line L132 (-4, -125.6967) -> (-1, -127.4287)
  line L133 (-1.3, -127.602) -> (-4, -126.0431)
  line L134 (-4, -126.0431) -> (-6.7, -127.602)
  line L135 (-7, -130.8928) -> (-7, -127.4287)
  line L136 (-6.7, -127.602) -> (-6.7, -130.7196)
  line L137 (-1.3, -130.7196) -> (-1.3, -127.602)
  line L138 (-1, -127.4287) -> (-1, -130.8928)
  line L139 (-1, -130.8928) -> (-4, -132.6249)
  line L140 (-4, -132.2785) -> (-1.3, -130.7196)
  line L141 (-6.7, -130.7196) -> (-4, -132.2785)
  line L142 (-4, -132.6249) -> (-7, -130.8928)
  line L143 (56.7, -118.4412) -> (56.7, -121.5588) projected
  line L144 (56.7, -78.4412) -> (56.7, -81.5588) projected
  line L145 (54, -3.4641) -> (54, -8.872)
  line L146 (54, -8.0829) -> (54, -31.9171) projected
  line L147 (57, -41.7321) -> (54, -43.4641)
  line L148 (54, -43.4641) -> (51, -41.7321)
  line L149 (51.3, -41.5588) -> (54, -43.1177)
  line L150 (54, -43.1177) -> (56.7, -41.5588)
  line L151 (56.7, -41.5588) -> (56.7, -38.4412)
  line L152 (57, -38.2679) -> (57, -41.7321)
  line L153 (54, -36.5359) -> (57, -38.2679)
  line L154 (56.7, -38.4412) -> (54, -36.8823)
  line L155 (51, -38.2679) -> (54, -36.5359)
  line L156 (54, -36.8823) -> (51.3, -38.4412)
  line L157 (51.3, -41.5588) -> (51.3, -38.4412)
  line L158 (51, -41.7321) -> (51, -38.2679)
  line L159 (57, -81.7321) -> (54, -83.4641)
  line L160 (54, -83.4641) -> (51, -81.7321)
  line L161 (51.3, -81.5588) -> (54, -83.1177)
  line L162 (54, -83.1177) -> (56.7, -81.5588)
  line L163 (56.7, -81.5588) -> (56.7, -78.4412)
  line L164 (57, -78.2679) -> (57, -81.7321)
  line L165 (54, -76.5359) -> (57, -78.2679)
  line L166 (56.7, -78.4412) -> (54, -76.8823)
  line L167 (51, -78.2679) -> (54, -76.5359)
  line L168 (54, -76.8823) -> (51.3, -78.4412)
  line L169 (51.3, -81.5588) -> (51.3, -78.4412)
  line L170 (51, -81.7321) -> (51, -78.2679)
  line L171 (57, -121.7321) -> (54, -123.4641)
  line L172 (54, -123.4641) -> (51, -121.7321)
  line L173 (51.3, -121.5588) -> (54, -123.1177)
  line L174 (54, -123.1177) -> (56.7, -121.5588)
  line L175 (56.7, -121.5588) -> (56.7, -118.4412)
  line L176 (57, -118.2679) -> (57, -121.7321)
  line L177 (54, -116.5359) -> (57, -118.2679)
  line L178 (56.7, -118.4412) -> (54, -116.8823)
  line L179 (51, -118.2679) -> (54, -116.5359)
  line L180 (54, -116.8823) -> (51.3, -118.4412)
  line L181 (51.3, -121.5588) -> (51.3, -118.4412)
  line L182 (51, -121.7321) -> (51, -118.2679)
  line L183 (57, -161.7321) -> (54, -163.4641)
  line L184 (54, -163.4641) -> (51, -161.7321)
  line L185 (51.3, -161.5588) -> (54, -163.1177)
  line L186 (54, -163.1177) -> (56.7, -161.5588)
  line L187 (56.7, -161.5588) -> (56.7, -158.4412)
  line L188 (57, -158.2679) -> (57, -161.7321)
  line L189 (54, -156.5359) -> (57, -158.2679)
  line L190 (56.7, -158.4412) -> (54, -156.8823)
  line L191 (51, -158.2679) -> (54, -156.5359)
  line L192 (54, -156.8823) -> (51.3, -158.4412)
  line L193 (51.3, -161.5588) -> (51.3, -158.4412)
  line L194 (51, -161.7321) -> (51, -158.2679)
  point P0 (56.7, -120)
  point P1 (56.7, -80)
  dimension "d471" = 6
  dimension "d472" = 108
  dimension "d475" = 360
  dimension "d479" = 360
  dimension "d481" = 6
  dimension "d484" = 30
  dimension "d489" = 40
  dimension "d492" = 40
  constraints: 364 end point, 14 equal length, 5 vertical, 2 midpoint, 1 centre point, 1 coincident, 1 point on line, 348 other
  measures "d471" distance between parallel lines of L10 L13
  measures "d472" diameter of A0
  measures "d481" distance between parallel lines of L116 L113
  measures "d484" distance of L113.end L119.start
  measures "d489" distance of point (56.7, -120) point (56.7, -80)
  measures "d492" distance of L36.end L147.start
extrude "押し出し19" cut sketch "スケッチ34" against normal blind 32 contours L1 L4 L3 L6 A0 L14 L15 L10 L11 L12 L0 | A0 L12 L13 L14 L6 L8 L0 | L52 L53 L54 L55 L56 A0 L95 L94 L99 L98 L97 | A0 L97 L96 L95 L56 L57 L52 | L20 L21 L16 A0 L61 L60 L59 | A0 L59 L58 L63 L62 L61 L16 L17 L18 L19 L20 | L46 L47 L48 L49 L50 A0 L89 L88 L93 L92 L91 | A0 L91 L90 L89 L50 L51 L46 | L40 L41 L42 L43 L44 A0 L83 L82 L87 L86 L85 | A0 L85 L84 L83 L44 L45 L40 | L34 L35 L36 L37 L38 A0 L77 L76 L81 L80 L79 | A0 L79 L78 L77 L38 L39 L34 | L111 L112 L113 L114 L115 L116 | L119 L120 L126 L127 L130 L123 | L131 L132 L138 L139 L142 L135 | L147 L148 L158 L155 L153 L152 | L159 L160 L170 L167 L165 L164 | L171 L172 L182 L179 L177 L176 | L183 L184 L194 L191 L189 L188
sketch "スケッチ35" plane through (0, 0, 35) normal (0, 0, 1) x (1, 0, 0)
  line L0 (-10.1344, -30) -> (69.4228, -30)
  line L1 (69.4228, -30) -> (69.4228, -195.12)
  line L2 (69.4228, -195.12) -> (-10.1344, -195.12)
  line L3 (-10.1344, -195.12) -> (-10.1344, -30)
  line L4 (57, -38.2679) -> (57, -41.7321) projected
  line L5 (-1, -130.8928) -> (-4, -132.6249) projected
  line L6 (-4, -132.6249) -> (-7, -130.8928) projected
  line L7 (-7, -130.8928) -> (-7, -127.4287) projected
  line L8 (-7, -127.4287) -> (-4, -125.6967) projected
  line L9 (-4, -125.6967) -> (-1, -127.4287) projected
  line L10 (-1, -127.4287) -> (-1, -130.8928) projected
  line L11 (51, -38.2679) -> (54, -36.5359) projected
  line L12 (54, -36.5359) -> (57, -38.2679) projected
  line L13 (57, -38.2679) -> (57, -41.7321) projected
  line L14 (57, -41.7321) -> (54, -43.4641) projected
  line L15 (54, -43.4641) -> (51, -41.7321) projected
  line L16 (51, -41.7321) -> (51, -38.2679) projected
  line L17 (-40.6333, -35.7343) -> (-37.2872, -34.8377) projected
  line L18 (-37.2872, -34.8377) -> (-34.8377, -37.2872) projected
  line L19 (-34.8377, -37.2872) -> (-35.7343, -40.6333) projected
  line L20 (-35.7343, -40.6333) -> (-39.0803, -41.5298) projected
  line L21 (-39.0803, -41.5298) -> (-41.5298, -39.0803) projected
  line L22 (-41.5298, -39.0803) -> (-40.6333, -35.7343) projected
  line L23 (-54, 3.4641) -> (-51, 1.7321) projected
  line L24 (-51, 1.7321) -> (-51, -1.7321) projected
  line L25 (-51, -1.7321) -> (-54, -3.4641) projected
  line L26 (-54, -3.4641) -> (-57, -1.7321) projected
  line L27 (-57, -1.7321) -> (-57, 1.7321) projected
  line L28 (-57, 1.7321) -> (-54, 3.4641) projected
  line L29 (54, -3.4641) -> (51, -1.7321) projected
  line L30 (51, -1.7321) -> (51, 1.7321) projected
  line L31 (51, 1.7321) -> (54, 3.4641) projected
  line L32 (54, 3.4641) -> (57, 1.7321) projected
  line L33 (57, 1.7321) -> (57, -1.7321) projected
  line L34 (57, -1.7321) -> (54, -3.4641) projected
  line L35 (51, -158.2679) -> (54, -156.5359) projected
  line L36 (54, -156.5359) -> (57, -158.2679) projected
  line L37 (57, -158.2679) -> (57, -161.7321) projected
  line L38 (57, -161.7321) -> (54, -163.4641) projected
  line L39 (54, -163.4641) -> (51, -161.7321) projected
  line L40 (51, -161.7321) -> (51, -158.2679) projected
  line L41 (-4, -102.6249) -> (-7, -100.8928) projected
  line L42 (-7, -100.8928) -> (-7, -97.4287) projected
  line L43 (-7, -97.4287) -> (-4, -95.6967) projected
  line L44 (-4, -95.6967) -> (-1, -97.4287) projected
  line L45 (-1, -97.4287) -> (-1, -100.8928) projected
  line L46 (-1, -100.8928) -> (-4, -102.6249) projected
  line L47 (51, -78.2679) -> (54, -76.5359) projected
  line L48 (54, -76.5359) -> (57, -78.2679) projected
  line L49 (57, -78.2679) -> (57, -81.7321) projected
  line L50 (57, -81.7321) -> (54, -83.4641) projected
  line L51 (54, -83.4641) -> (51, -81.7321) projected
  line L52 (51, -81.7321) -> (51, -78.2679) projected
  line L53 (3.4641, 54) -> (1.7321, 51) projected
  line L54 (1.7321, 51) -> (-1.7321, 51) projected
  line L55 (-1.7321, 51) -> (-3.4641, 54) projected
  line L56 (-3.4641, 54) -> (-1.7321, 57) projected
  line L57 (-1.7321, 57) -> (1.7321, 57) projected
  line L58 (1.7321, 57) -> (3.4641, 54) projected
  line L59 (-35.7343, 40.6333) -> (-34.8377, 37.2872) projected
  line L60 (-34.8377, 37.2872) -> (-37.2872, 34.8377) projected
  line L61 (-37.2872, 34.8377) -> (-40.6333, 35.7343) projected
  line L62 (-40.6333, 35.7343) -> (-41.5298, 39.0803) projected
  line L63 (-41.5298, 39.0803) -> (-39.0803, 41.5298) projected
  line L64 (-39.0803, 41.5298) -> (-35.7343, 40.6333) projected
  line L65 (40.6333, 35.7343) -> (37.2872, 34.8377) projected
  line L66 (37.2872, 34.8377) -> (34.8377, 37.2872) projected
  line L67 (34.8377, 37.2872) -> (35.7343, 40.6333) projected
  line L68 (35.7343, 40.6333) -> (39.0803, 41.5298) projected
  line L69 (39.0803, 41.5298) -> (41.5298, 39.0803) projected
  line L70 (41.5298, 39.0803) -> (40.6333, 35.7343) projected
  line L71 (51, -118.2679) -> (54, -116.5359) projected
  line L72 (54, -116.5359) -> (57, -118.2679) projected
  line L73 (57, -118.2679) -> (57, -121.7321) projected
  line L74 (57, -121.7321) -> (54, -123.4641) projected
  line L75 (54, -123.4641) -> (51, -121.7321) projected
  line L76 (51, -121.7321) -> (51, -118.2679) projected
  line L77 (-4, -65.6967) -> (-1, -67.4287) projected
  line L78 (-1, -67.4287) -> (-1, -70.8928) projected
  line L79 (-1, -70.8928) -> (-4, -72.6249) projected
  line L80 (-4, -72.6249) -> (-7, -70.8928) projected
  line L81 (-7, -70.8928) -> (-7, -67.4287) projected
  line L82 (-7, -67.4287) -> (-4, -65.6967) projected
  arc A0 (-31.7905, -37.506) -> (-32.3081, -35.5741) centre (-33.7223, -36.9883) ccw projected
  line L83 (-32.3081, -35.5741) -> (-35.5741, -32.3081) projected
  arc A1 (-35.5741, -32.3081) -> (-37.506, -31.7905) centre (-36.9883, -33.7223) ccw projected
  line L84 (-37.506, -31.7905) -> (-41.32, -32.8125) projected
  arc A2 (-43.4468, -32.0683) -> (-41.32, -32.8125) centre (-41.8376, -30.8806) ccw projected
  arc A3 (-53.3972, -8.0458) -> (-43.4468, -32.0683) centre (0, 0) ccw projected
  arc A4 (-52.4196, -6.0157) -> (-53.3972, -8.0458) centre (-51.4196, -7.7478) ccw projected
  line L85 (-52.4196, -6.0157) -> (-49, -4.0415) projected
  arc A5 (-49, -4.0415) -> (-48, -2.3094) centre (-50, -2.3094) ccw projected
  line L86 (-48, -2.3094) -> (-48, 2.3094) projected
  arc A6 (-48, 2.3094) -> (-49, 4.0415) centre (-50, 2.3094) ccw projected
  line L87 (-49, 4.0415) -> (-52.4196, 6.0157) projected
  arc A7 (-53.3972, 8.0458) -> (-52.4196, 6.0157) centre (-51.4196, 7.7478) ccw projected
  arc A8 (-43.4468, 32.0683) -> (-53.3972, 8.0458) centre (0, 0) ccw projected
  arc A9 (-41.32, 32.8125) -> (-43.4468, 32.0683) centre (-41.8376, 30.8806) ccw projected
  line L88 (-41.32, 32.8125) -> (-37.506, 31.7905) projected
  arc A10 (-37.506, 31.7905) -> (-35.5741, 32.3081) centre (-36.9883, 33.7223) ccw projected
  line L89 (-35.5741, 32.3081) -> (-32.3081, 35.5741) projected
  arc A11 (-32.3081, 35.5741) -> (-31.7905, 37.506) centre (-33.7223, 36.9883) ccw projected
  line L90 (-31.7905, 37.506) -> (-32.8125, 41.32) projected
  arc A12 (-32.0683, 43.4468) -> (-32.8125, 41.32) centre (-30.8806, 41.8376) ccw projected
  arc A13 (-8.0458, 53.3972) -> (-32.0683, 43.4468) centre (0, 0) ccw projected
  arc A14 (-6.0157, 52.4196) -> (-8.0458, 53.3972) centre (-7.7478, 51.4196) ccw projected
  line L91 (-6.0157, 52.4196) -> (-4.0415, 49) projected
  arc A15 (-4.0415, 49) -> (-2.3094, 48) centre (-2.3094, 50) ccw projected
  line L92 (-2.3094, 48) -> (2.3094, 48) projected
  arc A16 (2.3094, 48) -> (4.0415, 49) centre (2.3094, 50) ccw projected
  line L93 (4.0415, 49) -> (6.0157, 52.4196) projected
  arc A17 (8.0458, 53.3972) -> (6.0157, 52.4196) centre (7.7478, 51.4196) ccw projected
  arc A18 (32.0683, 43.4468) -> (8.0458, 53.3972) centre (0, 0) ccw projected
  arc A19 (32.8125, 41.32) -> (32.0683, 43.4468) centre (30.8806, 41.8376) ccw projected
  line L94 (32.8125, 41.32) -> (31.7905, 37.506) projected
  arc A20 (31.7905, 37.506) -> (32.3081, 35.5741) centre (33.7223, 36.9883) ccw projected
  line L95 (32.3081, 35.5741) -> (35.5741, 32.3081) projected
  arc A21 (35.5741, 32.3081) -> (37.506, 31.7905) centre (36.9883, 33.7223) ccw projected
  line L96 (37.506, 31.7905) -> (41.32, 32.8125) projected
  arc A22 (43.4468, 32.0683) -> (41.32, 32.8125) centre (41.8376, 30.8806) ccw projected
  arc A23 (53.3972, 8.0458) -> (43.4468, 32.0683) centre (0, 0) ccw projected
  arc A24 (52.4196, 6.0157) -> (53.3972, 8.0458) centre (51.4196, 7.7478) ccw projected
  line L97 (52.4196, 6.0157) -> (49, 4.0415) projected
  arc A25 (49, 4.0415) -> (48, 2.3094) centre (50, 2.3094) ccw projected
  line L98 (48, 2.3094) -> (48, -2.3094) projected
  arc A26 (48, -2.3094) -> (49, -4.0415) centre (50, -2.3094) ccw projected
  line L99 (49, -4.0415) -> (53, -6.3509) projected
  arc A27 (54, -8.0829) -> (53, -6.3509) centre (52, -8.0829) ccw projected
  line L100 (54, -8.0829) -> (54, -31.9171) projected
  arc A28 (53, -33.6491) -> (54, -31.9171) centre (52, -31.9171) ccw projected
  line L101 (53, -33.6491) -> (49, -35.9585) projected
  arc A29 (49, -35.9585) -> (48, -37.6906) centre (50, -37.6906) ccw projected
  line L102 (48, -37.6906) -> (48, -42.3094) projected
  arc A30 (48, -42.3094) -> (49, -44.0415) centre (50, -42.3094) ccw projected
  line L103 (49, -44.0415) -> (53, -46.3509) projected
  arc A31 (54, -48.0829) -> (53, -46.3509) centre (52, -48.0829) ccw projected
  line L104 (54, -48.0829) -> (54, -71.9171) projected
  arc A32 (53, -73.6491) -> (54, -71.9171) centre (52, -71.9171) ccw projected
  line L105 (53, -73.6491) -> (49, -75.9585) projected
  arc A33 (49, -75.9585) -> (48, -77.6906) centre (50, -77.6906) ccw projected
  line L106 (48, -77.6906) -> (48, -82.3094) projected
  arc A34 (48, -82.3094) -> (49, -84.0415) centre (50, -82.3094) ccw projected
  line L107 (49, -84.0415) -> (53, -86.3509) projected
  arc A35 (54, -88.0829) -> (53, -86.3509) centre (52, -88.0829) ccw projected
  line L108 (54, -88.0829) -> (54, -111.9171) projected
  arc A36 (53, -113.6491) -> (54, -111.9171) centre (52, -111.9171) ccw projected
  line L109 (53, -113.6491) -> (49, -115.9585) projected
  arc A37 (49, -115.9585) -> (48, -117.6906) centre (50, -117.6906) ccw projected
  line L110 (48, -117.6906) -> (48, -122.3094) projected
  arc A38 (48, -122.3094) -> (49, -124.0415) centre (50, -122.3094) ccw projected
  line L111 (49, -124.0415) -> (53, -126.3509) projected
  arc A39 (54, -128.0829) -> (53, -126.3509) centre (52, -128.0829) ccw projected
  line L112 (54, -128.0829) -> (54, -151.9171) projected
  arc A40 (53, -153.6491) -> (54, -151.9171) centre (52, -151.9171) ccw projected
  line L113 (53, -153.6491) -> (49, -155.9585) projected
  arc A41 (49, -155.9585) -> (48, -157.6906) centre (50, -157.6906) ccw projected
  line L114 (48, -157.6906) -> (48, -162.3094) projected
  arc A42 (48, -162.3094) -> (49, -164.0415) centre (50, -162.3094) ccw projected
  line L115 (49, -164.0415) -> (53, -166.3509) projected
  arc A43 (53, -166.3509) -> (55, -166.3509) centre (54, -164.6188) ccw projected
  line L116 (55, -166.3509) -> (59, -164.0415) projected
  arc A44 (59, -164.0415) -> (60, -162.3094) centre (58, -162.3094) ccw projected
  line L117 (60, -162.3094) -> (60, 0) projected
  arc A45 (60, 0) -> (-13.8462, -58.3805) centre (0, 0) ccw projected
  arc A46 (-10, -63.2456) -> (-13.8462, -58.3805) centre (-15, -63.2456) ccw projected
  line L118 (-10, -63.2456) -> (-10, -131.4702) projected
  arc A47 (-10, -131.4702) -> (-9, -133.2022) centre (-8, -131.4702) ccw projected
  line L119 (-9, -133.2022) -> (-5, -135.5117) projected
  arc A48 (-5, -135.5117) -> (-3, -135.5117) centre (-4, -133.7796) ccw projected
  line L120 (-3, -135.5117) -> (1, -133.2022) projected
  arc A49 (1, -133.2022) -> (2, -131.4702) centre (0, -131.4702) ccw projected
  line L121 (2, -131.4702) -> (2, -126.8514) projected
  arc A50 (2, -126.8514) -> (1, -125.1193) centre (0, -126.8514) ccw projected
  line L122 (1, -125.1193) -> (-3, -122.8099) projected
  arc A51 (-4, -121.0779) -> (-3, -122.8099) centre (-2, -121.0779) ccw projected
  line L123 (-4, -121.0779) -> (-4, -107.2437) projected
  arc A52 (-3, -105.5117) -> (-4, -107.2437) centre (-2, -107.2437) ccw projected
  line L124 (-3, -105.5117) -> (1, -103.2022) projected
  arc A53 (1, -103.2022) -> (2, -101.4702) centre (0, -101.4702) ccw projected
  line L125 (2, -101.4702) -> (2, -96.8514) projected
  arc A54 (2, -96.8514) -> (1, -95.1193) centre (0, -96.8514) ccw projected
  line L126 (1, -95.1193) -> (-3, -92.8099) projected
  arc A55 (-4, -91.0779) -> (-3, -92.8099) centre (-2, -91.0779) ccw projected
  line L127 (-4, -91.0779) -> (-4, -77.2437) projected
  arc A56 (-3, -75.5117) -> (-4, -77.2437) centre (-2, -77.2437) ccw projected
  line L128 (-3, -75.5117) -> (1, -73.2022) projected
  arc A57 (1, -73.2022) -> (2, -71.4702) centre (0, -71.4702) ccw projected
  line L129 (2, -71.4702) -> (2, -66.8514) projected
  arc A58 (2, -66.8514) -> (1, -65.1193) centre (0, -66.8514) ccw projected
  line L130 (1, -65.1193) -> (-3, -62.8099) projected
  arc A59 (-4, -61.0779) -> (-3, -62.8099) centre (-2, -61.0779) ccw projected
  line L131 (-4, -61.0779) -> (-4, -58.3095) projected
  arc A60 (-4, -58.3095) -> (-8.2373, -53.368) centre (-9, -58.3095) ccw projected
  arc A61 (-32.0683, -43.4468) -> (-8.2373, -53.368) centre (0, 0) ccw projected
  arc A62 (-32.8125, -41.32) -> (-32.0683, -43.4468) centre (-30.8806, -41.8376) ccw projected
  line L132 (-32.8125, -41.32) -> (-31.7905, -37.506) projected
  line L133 (-13.8462, -58.3805) -> (-12.2925, -52.5823)
  arc A63 (-32.0683, -43.4468) -> (-8.2373, -53.368) centre (0, 0) ccw projected
  point P0 (57, -40)
  point P1 (54, -140.235)
  point P2 (60, -140.235)
  point P3 (60, -30)
  point P4 (54, -30)
  point P5 (-10.1344, -62.0941)
  dimension "d499" = 10
  constraints: 10 end point, 2 parallel, 1 horizontal, 1 midpoint, 1 perpendicular, 1 point on circle
  measures "d499" distance from line of point (57, -40) L0
extrude "押し出し20" cut sketch "スケッチ35" against normal through all contours L0 L117 A44 L116 A43 L115 A42 L114 A41 L113 A40 L112 A39 L111 A38 L110 A37 L109 A36 L108 A35 L107 A34 L106 A33 L105 A32 L104 A31 L103 A30 L102 A29 L101 A28 L100 | A61 A60 L131 A59 L130 A58 L129 A57 L128 A56 L127 A55 L126 A54 L125 A53 L124 A52 L123 A51 L122 A50 L121 A49 L120 A48 L119 A47 L118 A46 L3 | L3 A46 L133 A61
fillet "フィレット18" radius 2 4 edges at (-12.2925, -52.5823, 20) (-13.8462, -58.3805, 20) (54, -30, 20) (60, -30, 20)
equation "\"d25\" = d24"
equation "\"d90\" = d89"
